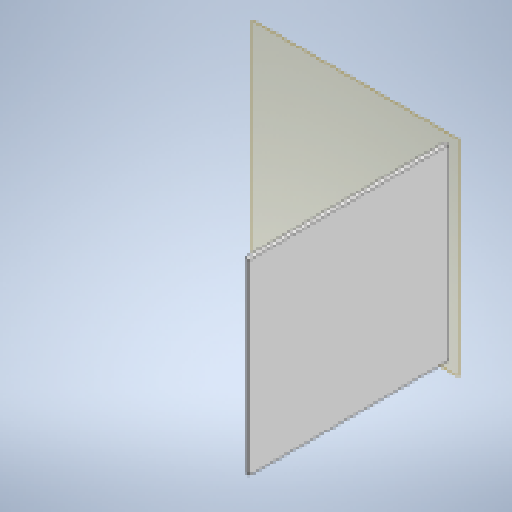
# Autodesk Inventor part: AcrilicoX
Saved by Autodesk Inventor 2024 (Build 280153000, 153)
## iProperties
Created: 2023-06-26
Part Number: AcrilicoX
Material: Genérico
Document SubType Name: Modeling
Designer: Personal
Density: 1.07292 g/cm^3
Appearance: Valor por defecto
Mass: 191.11 g
Surface Area: 845.069 cm^2
Volume: 178.121 cm^3
Author: Personal
Autodesk Inventor part; units mm, degrees
ref_plane "YZ Plane" through (0, 0, 0) normal (1, 0, 0) x (0, 1, 0)
ref_plane "XZ Plane" through (0, 0, 0) normal (0, 1, 0) x (-1, 0, 0)
ref_plane "Plano de trabajo1" through (0, 0, 0) normal (0, 0, 1) x (1, 0, 0)
sketch "Boceto1" plane through (0, 0, 0) normal (0, 0, 1) x (1, 0, 0)
  line L0 (97.5, -97.5) -> (97.5, 97.5) construction
  line L1 (93.1, -97.5) -> (97.5, -97.5)
  line L2 (97.5, -97.5) -> (97.5, 97.5)
  line L3 (97.5, 97.5) -> (93.1, 97.5)
  line L4 (93.1, 97.5) -> (93.1, -97.5)
  point P0 (0, 0)
  dimension "d0" = 195
  dimension "d1" = 4.4
  constraints: 8 end point, 2 parallel, 1 horizontal, 1 perpendicular
  measures "d0" distance of L3.end L1.start
  measures "d1" distance between parallel lines of L0 L4
extrude "Extrusión1" add sketch "Boceto1" along normal blind 207.6
